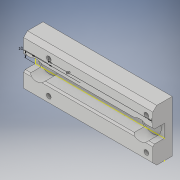
# Autodesk Inventor part: pcb_x_carriage_addon
Saved by Autodesk Inventor 2019 (Build 230136000, 136)
## iProperties
Created: 2020-04-21
Part Number: pcb_x_carriage_addon
Material: Generisch
Document SubType Name: Modeling
Designer: marc
Density: 1 g/cm^3
Appearance: Vorgabe
Author: marc
## iProperties of the stored document pcb_x_carriage_addon_3D-Druck.ipt
Created: 2020-04-21
Part Number: pcb_x_carriage_addon_3D-Druck
Material: Generisch
Document SubType Name: Modeling
Designer: marc
Density: 1 g/cm^3
Appearance: Vorgabe
Author: marc
Autodesk Inventor part; units mm, degrees
ref_plane "YZ Plane" through (0, 0, 0) normal (1, 0, 0) x (0, 1, 0)
ref_plane "XZ Plane" through (0, 0, 0) normal (0, 1, 0) x (-1, 0, 0)
ref_plane "XY Plane" through (0, 0, 0) normal (0, 0, 1) x (1, 0, 0)
sketch "Skizze1" plane through (0, 0, 0) normal (0, 0, 1) x (1, 0, 0)
  line L0 (0, 0) -> (-100, 0)
  line L1 (-100, 0) -> (-100, 40)
  line L2 (-100, 40) -> (0, 40)
  line L3 (0, 40) -> (0, 0)
  dimension "d0" = 100
  dimension "d1" = 40
  constraints: 8 end point, 2 parallel, 1 horizontal, 1 perpendicular
  measures "d0" distance of L1.end L2.end
  measures "d1" distance of L0.end L1.end
extrude "Extrusion1" add sketch "Skizze1" along normal blind 15
sketch "Skizze2" plane through (0, 0, 15) normal (0, 0, 1) x (1, 0, 0)
  line L0 (-100, 40) -> (-100, 0) projected
  line L1 (-100, 25) -> (0, 25)
  line L2 (0, 25) -> (0, 15)
  line L3 (0, 15) -> (-100, 15)
  line L4 (-100, 15) -> (-100, 25)
  line L5 (0, 40) -> (-100, 40) projected
  line L6 (-100, 0) -> (0, 0) projected
  line L7 (0, 0) -> (0, 40) projected
  dimension "d4" = 15
  dimension "d5" = 15
  constraints: 8 end point, 2 parallel, 2 point on line, 1 horizontal, 1 perpendicular
  measures "d4" distance between parallel lines of L5 L1
  measures "d5" distance between parallel lines of L6 L3
extrude "Extrusion2" cut sketch "Skizze2" against normal blind 9 contours L1 L2 L3 L0
sketch "Skizze3" plane through (0, 0, 15) normal (0, 0, 1) x (1, 0, 0)
  line L0 (0, 0) -> (0, 15) projected
  line L1 (-100, 0) -> (0, 0) projected
  line L2 (-100, 25) -> (0, 25) projected
  point P0 (-5, 32.5)
  point P1 (-80.5, 32.5)
  point P2 (-5, 7.5)
  point P3 (-80.5, 7.5)
  dimension "d8" = 75.5
  dimension "d9" = 5
  dimension "d10" = 7.5
  dimension "d11" = 7.5
  constraints: 2 horizontal alignment, 2 vertical alignment
  measures "d8" distance of point (-80.5, 7.5) point (-5, 7.5)
  measures "d9" distance from line of L0 point (-5, 7.5)
  measures "d10" distance from line of L1 point (-5, 7.5)
  measures "d11" distance from line of L2 point (-5, 32.5)
hole "Bohrung1" at (-5, 32.5, 15) at (-80.5, 32.5, 15) at (-5, 7.5, 15) at (-80.5, 7.5, 15) direction (0, 0, -1) diameter 3.6 end through all clearance for "Flachkopfsenkschraube DIN EN ISO 2009" size "M3" standard "DIN"
sketch "Skizze4" plane through (0, 0, 6) normal (0, 0, 1) x (1, 0, 0)
  line L0 (-100, 15) -> (-100, 25) projected
  line L1 (0, 15) -> (-100, 15) projected
  point P0 (0, 0)
  point P1 (-10, 20)
  point P2 (-90, 20)
  dimension "d19" = 80
  dimension "d20" = 10
  dimension "d21" = 5
  constraints: 1 horizontal alignment
  measures "d19" distance of point (-90, 20) point (-10, 20)
  measures "d20" distance from line of L0 point (-90, 20)
  measures "d21" distance from line of L1 point (-90, 20)
hole "Bohrung2" at (-10, 20, 6) at (-90, 20, 6) direction (0, 0, -1) diameter 5.8 end through all counterbore diameter 15 counterbore depth 1 clearance for "Sechskantkopfschraube DIN EN 24017" size "M5" standard "DIN"
hole "Bohrung3" at (-10, 20, 6) at (-90, 20, 6) direction (0, 0, 1) diameter 15 end through all
chamfer "Fase1" distance 3 angle 45 2 edges at (-50, 0, 15) (-50, 40, 15)
chamfer "Fase2" distance 1.25 angle 45 6 edges at (-97.7951, 25, 15) (-2.2049, 25, 15) (-50, 25, 15) (-97.7951, 15, 15) (-2.2049, 15, 15) (-50, 15, 15)
equation "\"d11\" = d10"
